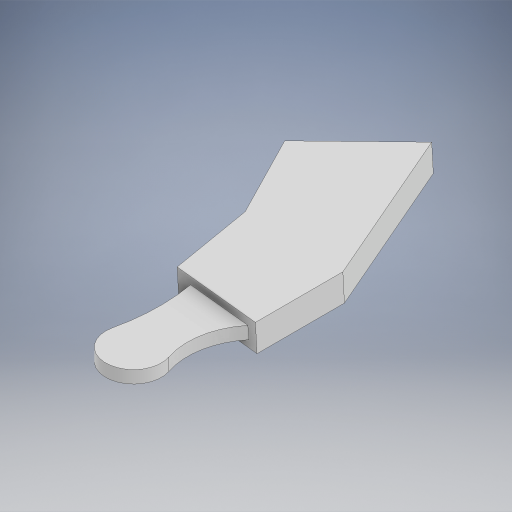
# Autodesk Inventor part: brace2.0
Saved by Autodesk Inventor 2024 (Build 280153000, 153)
## iProperties
Created: 2024-12-18
Part Number: brace2.0
Material: Generic
Document SubType Name: Modeling
Designer: Alex
Density: 1 g/cm^3
Appearance: Default
Author: Alex
Autodesk Inventor part; units mm, degrees
ref_plane "YZ Plane" through (0, 0, 0) normal (1, 0, 0) x (0, 1, 0)
ref_plane "XY Plane" through (0, 0, 0) normal (0, 0, 1) x (1, 0, 0)
sketch "Sketch1" plane through (0, 0, 0) normal (0, 1, 0) x (-1, 0, 0)
  circle A0 centre (0, 0) radius 10
  line L0 (10, 0) -> (9.2097, -30.1236) construction
  arc A1 (-17.027, -27.0939) -> (14.3169, -30.2866) centre (17.8178, 159.5407) ccw construction
  line L1 (0, 0) -> (-14.0737, -27.6212) construction
  line L2 (10, 0) -> (-10, 0) construction
  line L3 (0, -10) -> (0, 10) construction
  arc A2 (9.7489, -2.227) -> (9.2097, -30.1236) centre (76.4766, -17.4702) ccw
  arc A3 (-14.0737, -27.6212) -> (-9.4804, -3.1816) centre (-33.645, -11.2914) ccw
  line L4 (0, 0) -> (9.2097, -30.1236) construction
  line L5 (14.3169, -30.2866) -> (-17.027, -27.0939) construction
  line L6 (9.2097, -30.1236) -> (-14.0737, -27.6212) construction
  line L7 (-1.355, -28.6902) -> (-1.4214, -29.3415) construction
  line L8 (0, 0) -> (-17.027, -27.0939) construction
  line L9 (0, 0) -> (14.3169, -30.2866) construction
  line L10 (-17.027, -27.0939) -> (-14.0737, -27.6212) construction
  line L11 (0, 0) -> (-18.5691, -57.0543) construction
  line L12 (0, 0) -> (17.8587, -58.3272) construction
  line L13 (17.8587, -58.3272) -> (-18.5691, -57.0543) construction
  line L14 (-18.5691, -57.0543) -> (-17.027, -27.0939) construction
  line L15 (14.3169, -30.2866) -> (17.8587, -58.3272) construction
  line L16 (14.3169, -30.2866) -> (17.8587, -58.3272) construction
  line L17 (-17.027, -27.0939) -> (-18.5691, -57.0543) construction
  line L18 (17.8587, -58.3272) -> (31.4475, -86.1902) construction
  line L19 (-18.5691, -57.0543) -> (3.1581, -110.8309) construction
  line L20 (-18.5691, -57.0543) -> (39.4309, -57.0543) construction
  arc A4 (17.8587, -58.3272) -> (31.4475, -86.1902) centre (65.5771, -52.3) ccw construction
  arc A5 (-18.5691, -57.0543) -> (3.1581, -110.8309) centre (50.0978, -60.5886) ccw construction
  line L21 (31.4475, -86.1902) -> (3.1581, -110.8309) construction
  arc A6 (-14.0737, -27.6212) -> (9.2097, -30.1236) centre (17.8178, 159.5407) ccw
  dimension "d0" = 20
  dimension "d4" = 63
  dimension "d7" = 31
  dimension "d8" = 73
  dimension "d9" = 31.5
  dimension "d14" = 32
  dimension "d15" = 33.5
  dimension "d19" = 3
  dimension "d20" = 60
  dimension "d21" = 61
  dimension "d22" = 36.45
  dimension "d23" = 30
  dimension "d24" = 68.4466
  dimension "d25" = 25.4892
  dimension "d26" = 118
  dimension "d27" = 31
  dimension "d28" = 58
  dimension "d29" = 68
  dimension "d30" = 37.5161
  dimension "d142" = 28.2635
  dimension "d149" = 87.13
  dimension "d150" = 103.015
  dimension "d152" = 65.999
  constraints: 44 end point, 21 point on circle, 7 centre point, 4 tangent, 2 collinear, 2 horizontal, 1 coincident, 1 concentric, 1 equal length, 1 midpoint, 1 vertical
  measures "d0" diameter of A0
  measures "d4" angle of L2 L1
  measures "d7" distance of L1.start L1.end
  measures "d8" angle of L2 L4
  measures "d9" distance of L1.start L0.end
  measures "d14" distance of L1.start L5.end
  measures "d15" distance of L1.start L5.start
  measures "d19" distance of L5.end L1.end
  measures "d20" distance of L1.start L11.end
  measures "d21" distance of L1.start L12.end
  measures "d22" distance of L12.end L11.end
  measures "d23" distance of L11.end L5.end
  measures "d24" radius of A2
  measures "d25" radius of A3
  measures "d26" angle of L13 L18
  measures "d27" distance of L12.end L18.end
  measures "d28" distance of L11.end L19.end
  measures "d29" angle of L19 L20
  measures "d30" distance of L18.end L19.end
  measures "d142" distance of L5.start L12.end
  measures "d149" angle of L14 L5
  measures "d150" angle of L5 L15
  measures "d152" angle of L19 L13
ref_plane "Work Plane11" through (-14.3169, 0, -30.2866) normal (-0.0053, 0.9986, 0.0521) x (0.9949, 0, 0.1013)
sketch "Sketch9" plane through (-14.3169, 0, -30.2866) normal (-0.0053, 0.9986, 0.0521) x (0.9949, 0, 0.1013)
  line L0 (0, 0) -> (31.5061, 0) projected
  line L1 (31.5061, 0) -> (30.004, 29.9624)
  line L2 (0, 0) -> (-6.3652, 27.5369)
  line L3 (-6.3652, 27.5369) -> (30.004, 29.9624) construction
  line L4 (-6.3652, 27.5369) -> (-22.7067, 53.88)
  line L5 (-22.7067, 53.88) -> (2.9398, 81.2608)
  line L6 (2.9398, 81.2608) -> (30.004, 29.9624)
  point P0 (17.3123, -28.6406)
  dimension "d141" = 30
  dimension "d143" = 28.263
  dimension "d144" = 36.45
  dimension "d146" = 58
  dimension "d147" = 31
  dimension "d148" = 37.516
  dimension "d151" = 87.13
  dimension "d153" = 66
  constraints: 12 end point
  measures "d141" distance of L0.end L1.end
  measures "d143" distance of L0.start L2.end
  measures "d144" distance of L2.end L1.end
  measures "d146" distance of L5.end L1.end
  measures "d147" distance of L2.end L4.end
  measures "d148" distance of L4.end L5.end
  measures "d151" angle of L0 L1
  measures "d153" angle of L6 L3
extrude "Extrusion6" add sketch "Sketch1" along normal mid plane 4.5
extrude "Extrusion7" add sketch "Sketch9" along normal mid plane 10
body "Solid2"
